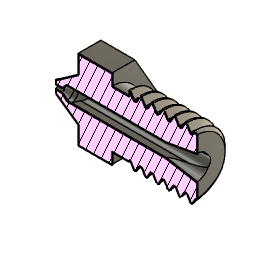
E3D Hi-Flow Nozzle v3 (Autodesk Fusion 360 design; units mm, degrees)
Autodesk Fusion 360 part; units mm, degrees
sketch "Sketch1" plane through (0, 0, 0) normal (0, 0, 1) x (1, 0, 0)
  line L0 (0, 3) -> (-6, 3)
  line L1 (-6, 3) -> (-6, 2.5)
  line L2 (-6, 2.5) -> (-7.5, 2.5)
  line L3 (-7.5, 2.5) -> (-7.5, 4.05)
  line L4 (-7.5, 4.05) -> (-10.5, 4.05)
  line L5 (-10.5, 4.05) -> (-10.5, 1.9004)
  line L6 (-10.5, 1.9004) -> (-12.5, 0.5)
  line L7 (-12.5, 0.5) -> (-12.5, 0)
  line L8 (-12.5, 0) -> (0, 0)
  line L9 (0, 3) -> (0, 0)
  line L10 (-7.5, -4.05) -> (-10.5, -4.05)
  line L11 (0, -3) -> (-6, -3)
  line L12 (-10.5, -4.05) -> (-10.5, -1.9004)
  line L13 (-7.5, -2.5) -> (-7.5, -4.05)
  line L14 (-6, -3) -> (-6, -2.5)
  line L15 (-10.5, -1.9004) -> (-12.5, -0.5)
  line L16 (-6, -2.5) -> (-7.5, -2.5)
  line L17 (0, -3) -> (0, 0)
  line L18 (-12.5, -0.5) -> (-12.5, 0)
  line L19 (-0.5, -3) -> (0, -2.5)
  dimension "d1" = 6
  dimension "d2" = 7.5
  dimension "d3" = 3
  dimension "d4" = 6
  dimension "d5" = 5
  dimension "d6" = 5
  dimension "d7" = 35
  dimension "d8" = 1
  dimension "d9" = 8.1
  dimension "d17" = 45
  dimension "d18" = 0.5
  constraint horizontal L0
  constraint perpendicular L0 L1
  constraint perpendicular L1 L2
  constraint perpendicular L2 L3
  constraint perpendicular L3 L4
  constraint perpendicular L4 L5
  constraint perpendicular L4 L7
  constraint coincident L8.end L9.end
  constraint vertical L9
  constraint horizontal L8
  constraint symmetric L0.start L8 L11.start
  constraint symmetric L0.end L8 L11.end
  constraint symmetric L1.end L8 L14.end
  constraint symmetric L2.end L8 L13.start
  constraint symmetric L3.end L8 L10.start
  constraint symmetric L4.end L8 L10.end
  constraint symmetric L5.end L8 L12.end
  constraint symmetric L6.end L8 L15.end
  constraint symmetric L7.end L8 L18.end
  constraint symmetric L9.end L8 L17.end
  constraint coincident L0.start L9.start
  constraint coincident L11 L19.start
  constraint coincident L17 L19.end
  measures "d1" distance of L1 L9
  measures "d2" distance of L3 L9
  measures "d3" distance of L3.end L4.end
  measures "d6" distance of L3 L7
  measures "d7" angle of L6 L8
  measures "d17" angle of L17 L19
  measures "d18" distance of L11.start L19.start
revolve "Revolve1" add sketch "Sketch1" angle 360 about axis through (-12.5, 0, 0) along (1, 0, 0) contours L0 L1 L2 L3 L4 L5 L6 L7 L8 L9
sketch "Sketch2" plane through (0, 0, 0) normal (1, 0, 0) x (0, 1, 0)
  line L0 (-2.0207, 3.5) -> (-4.0415, 0)
  line L1 (-4.0415, 0) -> (-2.0207, -3.5)
  line L2 (-2.0207, -3.5) -> (2.0207, -3.5)
  line L3 (2.0207, -3.5) -> (4.0415, 0)
  line L4 (4.0415, 0) -> (2.0207, 3.5)
  line L5 (2.0207, 3.5) -> (-2.0207, 3.5)
  dimension "d14" = 7
  constraint horizontal L5
  measures "d14" distance of L2 L5
extrude "Extrude1" cut sketch "Sketch2" against normal up to surface (12.5 mm away) keep common part
thread "Thread1" "ISO Metric profile 6.0 M6x1 6g" major diameter 5.884 minor diameter 4.7435 pitch 1 angle 60 modelled right hand crest width 0.1444 on face at (-2, 2.9963, -0.1495) crest through (-6.25, 2.942, 0)
revolve "Revolve2" cut sketch "Sketch1" angle 360 about axis through (-12.5, 0, 0) along (1, 0, 0) contours L11 L17 L19
sketch "Sketch3" plane through (0, 0, 0) normal (1, 0, 0) x (0, 1, 0)
  circle A0 centre (0, 0) radius 0.2
  circle A1 centre (0, 0) radius 0.6125
  circle A2 centre (0, 0) radius 1.0938
  line L0 (-0.5989, 0.6125) -> (0.5989, 0.6125)
  line L1 (-0.5989, -0.6125) -> (0.5989, -0.6125)
  arc A3 (-0.5989, 0.6125) -> (-0.5989, -0.6125) centre (-0.5989, 0) ccw
  arc A4 (0.5989, -0.6125) -> (0.5989, 0.6125) centre (0.5989, 0) ccw
  dimension "d20" = 0.4
  dimension "d24" = 1.225
  dimension "d26" = 2.1875
  dimension "d27" = 1.1977
  dimension "d29" = 0.5989
  constraint coincident A0.centre A1.centre
  constraint tangent L0 A4
  constraint tangent L1 A4
  constraint tangent L0 A3
  constraint tangent L1 A3
  constraint horizontal A0.centre A3.centre
  constraint horizontal A0.centre A4.centre
  constraint equal A1 A3
  constraint equal A1 A4
  measures "d20" diameter of A0
  measures "d24" diameter of A1
  measures "d26" diameter of A2
  measures "d27" distance of A3.centre A4.centre
  measures "d29" distance of A0.centre A3.centre
extrude "Extrude2" cut sketch "Sketch3" against normal through all contours A0
extrude "Extrude3" cut sketch "Sketch3" against normal up to surface (11.5 mm away) contours A1
extrude "Extrude4" cut sketch "Sketch3" against normal up to surface (10.5 mm away) contours A0 | A1 | A1 A2 L0 L1 A4 | A1 A2 L0 L1 A3 | A2 A3 | A2 A4
extrude "Extrude5" cut sketch "Sketch3" against normal blind 10 draft -10 contours A0 | A1 | A1 A2 L0 L1 A4 | A1 A2 L0 L1 A3 | A2 L0 A3 A4 | A2 L1 A3 A4
chamfer "Chamfer1" distance 0.4125 angle 45 1 edges at (-11.5, -0.1865, -0.0723)
chamfer "Chamfer2" distance 0.5988 angle 45 2 edges at (-10.5, -0.6125, 0) (-10.5, 0.6125, 0)
equation "d8 = Nozzle_d + 0.6 mm"
equation "Nozzle_d = 0.4 mm"
equation "d20 = Nozzle_d"
equation "filament = 1.75 mm"
equation "enlarge = 1.25"
equation "d24 = filament * push"
equation "push = 0.7"
equation "d26 = filament * enlarge"
equation "d27 = width"
equation "d29 = d27 / 2"
equation "d37 = filament * push / 2 - Nozzle_d / 2"
equation "d38 = width / 2 - 0.0001 mm"
equation "K_factor = 1.1"
equation "width = PI * filament / 4 * ( K_factor / push - push )"
